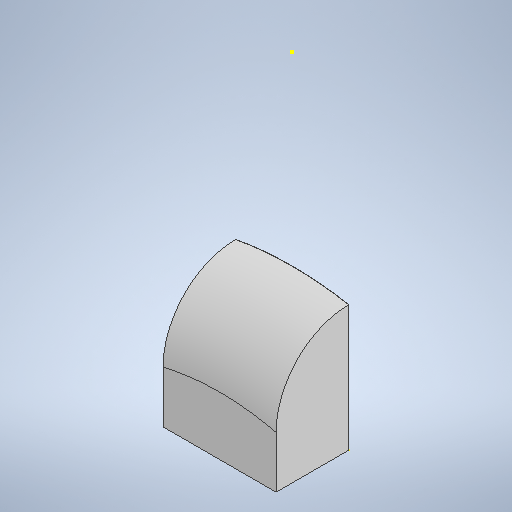
# Autodesk Inventor part: thermal camera lid
Saved by Autodesk Inventor 2025.2 (Build 292293000, 293)
## iProperties
Created: 2025-08-14
Part Number: thermal camera lid
Material: Generic
Document SubType Name: Modeling
Designer: mateo
Density: 1 g/cm^3
Appearance: Default
Author: mateo
Autodesk Inventor part; units mm, degrees
ref_plane "YZ Plane" through (0, 0, 0) normal (1, 0, 0) x (0, 1, 0)
ref_plane "XZ Plane" through (0, 0, 0) normal (0, 1, 0) x (-1, 0, 0)
ref_plane "XY Plane" through (0, 0, 0) normal (0, 0, 1) x (1, 0, 0)
sketch "Sketch1" plane through (0, 0, 0) normal (0, 0, 1) x (1, 0, 0)
  line L0 (-34.925, -117.475) -> (-34.925, -195.2625)
  line L1 (-34.925, -195.2625) -> (34.925, -195.2625)
  line L2 (34.925, -195.2625) -> (34.925, -117.475)
  arc A0 (34.925, -117.475) -> (-34.925, -117.475) centre (0, -307.975) ccw
  point P0 (0, 0)
  constraints: 6 end point, 2 point on circle, 1 centre point, 1 parallel
extrude "Extrusion1" add sketch "Sketch1" along normal blind 45
fillet "Fillet1" radius 44.8625 1 edges at (0, -114.3, 45)
shell "Shell1" thickness 6 removed faces 1 at (0, -168.275, 0)
sketch "Sketch4" plane through (-34.925, -195.2625, 0) normal (0, -1, 0) x (1, 0, 0)
  line L0 (6, 0) -> (6, 39) projected
  line L1 (63.8503, 0) -> (63.8503, -45) projected
  line L2 (6, 39) -> (63.8503, 39)
  line L3 (63.8503, 39) -> (63.8503, -6.35)
  line L4 (63.8503, -6.35) -> (6, -6.35)
  line L5 (6, -6.35) -> (6, 39)
  point P0 (34.925, 0)
  constraints: 8 end point, 2 parallel, 1 horizontal, 1 perpendicular, 1 point on line
extrude "Extrusion3" cut sketch "Sketch4" against normal blind 6
sketch "Sketch5" plane through (0, 0, 0) normal (0, 0, -1) x (-1, 0, 0)
  line L0 (28.925, -122.5424) -> (28.925, -195.2625) projected
  line L1 (28.925, -149.5135) -> (28.925, -147.6375)
  line L2 (34.925, -195.2625) -> (28.925, -195.2625) projected
  line L3 (-28.925, -141.9835) -> (-32.925, -149.5135)
  line L4 (-32.925, -149.5135) -> (-28.925, -149.5135)
  line L5 (-28.925, -141.9835) -> (-28.925, -149.5135)
  line L6 (-28.9253, -195.2625) -> (-34.925, -195.2625) projected
  line L7 (-28.925, -189.2625) -> (-28.925, -122.5424) projected
  line L8 (28.925, -141.9835) -> (28.925, -149.5135)
  line L9 (32.925, -149.5135) -> (28.925, -149.5135)
  line L10 (28.925, -141.9835) -> (32.925, -149.5135)
  point P0 (0, 0)
  constraints: 14 end point, 2 point on line
body "Solid1"
